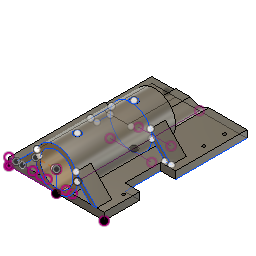
Pen Holder v2 (Autodesk Fusion 360 design; units mm, degrees)
Autodesk Fusion 360 part; units mm, degrees
sketch "Sketch1" plane through (0, 0, 0) normal (0, 1, 0) x (1, 0, 0)
  line L0 (0, 0) -> (32, 0)
  line L1 (32, 0) -> (32, 12)
  line L2 (32, 12) -> (27, 12)
  line L3 (27, 12) -> (27, 24)
  line L4 (27, 24) -> (32, 24)
  line L5 (32, 24) -> (32, 48)
  line L6 (32, 48) -> (0, 48)
  line L7 (0, 48) -> (0, 0)
  line L8 (0, 48) -> (16, 48)
  line L9 (16, 48) -> (16, 0)
  line L10 (0, 48) -> (5, 48)
  line L11 (8, 48) -> (8, 32)
  line L12 (8, 32) -> (0, 32)
  dimension "d1" = 32
  dimension "d2" = 12
  dimension "d3" = 12
  dimension "d4" = 24
  dimension "d5" = 16
  dimension "d6" = 5
  dimension "d7" = 16
  constraint coincident L0.start L7.end
  constraint horizontal L0
  constraint perpendicular L0 L1
  constraint horizontal L2
  constraint perpendicular L2 L3
  constraint perpendicular L3 L4
  constraint perpendicular L4 L5
  constraint perpendicular L5 L6
  constraint perpendicular L0 L7
  constraint coincident L6 L8.end
  constraint midpoint L0 L9.end
  constraint perpendicular L7 L10
  constraint midpoint L8 L11.start
  constraint perpendicular L8 L11
  constraint coincident L7 L12.end
  constraint perpendicular L7 L12
  measures "d1" distance of L0.start L0.end
  measures "d2" distance of L0.end L1.end
  measures "d3" distance of L2.end L3.end
  measures "d4" distance of L4.end L5.end
  measures "d5" distance of L6.end L8.end
  measures "d6" distance of L6.end L10.end
  measures "d7" distance of L11.start L11.end
extrude "Extrude1" add sketch "Sketch1" along normal blind 2.5 contours L0 L6 L7 L8 L9 L11 L12 | L0 L1 L2 L3 L4 L5 L6 L9 makes body 1
extrude "Extrude2" add sketch "Sketch1" along normal blind 2 contours L6 L7 L8 L10 L11 L12 bodies 1
sketch "Sketch2" plane through (0, 0, 0) normal (0, 0, 1) x (1, 0, 0)
  line L0 (32, 0) -> (0, 0)
  line L1 (32, 0) -> (16, 0)
  line L2 (0, 0) -> (32, 0)
  line L3 (0, 0) -> (32, 0)
  circle A0 centre (16, 7) radius 5.5
  circle A1 centre (16, 7) radius 7
  point P0 (32, 0)
  dimension "d12" = 16
  dimension "d14" = 11
  constraint coincident P0 L0.start
  constraint parallel L0 L1
  measures "d12" distance of P0 L1.end
  measures "d14" diameter of A0
extrude "Extrude3" cut sketch "Sketch2" against normal blind 53 contours A0 bodies 1
extrude "Extrude4" add sketch "Sketch2" against normal blind 33 bodies 1
sketch "Sketch3" plane through (0, 0, 0) normal (0, 0, 1) x (1, 0, 0)
  circle A0 centre (16, 7) radius 7
  line L0 (8, 2.5) -> (0, 2.5)
  line L1 (9.0003, 6.936) -> (4.5642, 2.5)
  line L2 (9.0003, 6.936) -> (15.2738, 6.936) construction
  line L3 (9.4734, 9.5304) -> (2.4429, 2.5)
  line L4 (7.9396, 7.9967) -> (10.1087, 7.9967) construction
  arc A1 (12.8377, 2.5) -> (19.1623, 2.5) centre (16, 7) ccw
  line L5 (16, 7) -> (16, 1.5)
  line L6 (22.5266, 9.5304) -> (29.5571, 2.5)
  line L7 (22.9997, 6.936) -> (27.4358, 2.5)
  line L8 (29.5571, 2.5) -> (27.4358, 2.5)
  line L9 (9.4734, 9.5304) -> (2.4429, 2.5)
  line L10 (9.0003, 6.936) -> (4.5642, 2.5)
  line L11 (9.4734, 9.5304) -> (2.4429, 2.5)
  line L12 (9.0003, 6.936) -> (4.5642, 2.5)
  line L13 (22.9997, 6.936, -25) -> (27.4358, 2.5, -25)
  line L14 (22.5266, 9.5304, -25) -> (29.5571, 2.5, -25)
  line L15 (9.4734, 9.5304, -25) -> (2.4429, 2.5, -25)
  line L16 (9.0003, 6.936, -25) -> (4.5642, 2.5, -25)
  line L17 (4.5642, 2.5, -25) -> (2.452, 2.5091, -25)
  line L18 (29.5571, 2.5, -25) -> (27.4358, 2.5, -25)
  circle A2 through (23, 7, -25) (12.5, 13.0622, -25) (12.5, 0.9378, -25)
  arc A3 (21.3619, 2.5) -> (10.6381, 2.5) centre (16, 7) ccw
  constraint coincident A0 L1.start
  constraint coincident L0 L1.end
  constraint coincident L4.start L3
  constraint coincident L0 L3.end
  constraint coincident A0.centre A1.centre
  constraint midpoint A1 L5.end
extrude "Extrude5" add sketch "Sketch3" against normal blind 5 contours A0 L0 L1 L3 L9 L10 L11 L12 A3 bodies 1
extrude "Extrude6" add sketch "Sketch3" against normal blind 5 contours A0 L6 L7 L8 A3 bodies 1
extrude "Extrude7" add sketch "Sketch3" against normal blind 5 separate body contours L13 L14 L18 A2 | L15 L16 L17 A2 in plane through (0, 0, -25) normal (0, 0, 1) makes body 2 at (7.1329, 7.19, -26.6667) makes body 3 at (24.8701, 7.187, -26.6667)
sketch "Sketch4" plane through (0, 0, 0) normal (0, 1, 0) x (1, 0, 0)
  line L0 (16, 48) -> (16, 0)
  line L1 (16, 0) -> (16, 7)
  circle A0 centre (16, 7) radius 1.25
  line L2 (10.5, 33) -> (21.5, 33)
  line L3 (9, 25) -> (23, 25)
  line L4 (16, 33) -> (16, 26)
  circle A1 centre (16, 26) radius 1.25
  circle A2 through (17.25, 26, 14) (15.375, 27.0825, 14) (15.375, 24.9175, 14)
  circle A3 through (17.25, 7, 14) (15.375, 8.0825, 14) (15.375, 5.9175, 14)
  point P0 (16, 0)
  dimension "d30" = 7
  dimension "d31" = 2.5
  dimension "d32" = 7
  dimension "d33" = 2.5
  constraint coincident P0 L0.end
  constraint coincident L0 L1.end
  constraint coincident L1.end A0.centre
  constraint midpoint L2 L4.start
  constraint perpendicular L3 L4
  constraint coincident L4.end A1.centre
  measures "d30" distance of P0 L1.end
  measures "d31" diameter of A0
  measures "d32" distance of L4.start L4.end
  measures "d33" diameter of A1
extrude "Extrude8" cut sketch "Sketch4" against normal blind 3 contours A2 | A3 in plane through (0, 14, 0) normal (0, 1, 0) bodies 1
sketch "Sketch7" plane through (0, 2.5, 0) normal (0, 1, 0) x (-1, 0, 0)
  line L0 (-27.4358, 0) -> (-27.4358, -5)
  line L1 (-27.4358, -5) -> (-29.5571, -5)
  line L2 (-29.5571, -5) -> (-29.5571, 0)
  line L3 (-29.5571, 0) -> (-32, 0)
  line L4 (-32, 0) -> (-32, -12)
  line L5 (-32, -12) -> (-27, -12)
  line L6 (-27, -12) -> (-27, -24)
  line L7 (-27, -24) -> (-32, -24)
  line L8 (-32, -24) -> (-32, -48)
  line L9 (-32, -48) -> (-19.1623, -48)
  line L10 (-19.1623, -48) -> (-19.1623, -33)
  line L11 (-19.1623, -33) -> (-21.3619, -33)
  line L12 (-21.3619, -33) -> (-21.3619, 0)
  line L13 (-21.3619, 0) -> (-27.4358, 0)
  line L14 (-32, -48) -> (-29.5, -48)
  line L15 (-29.5, -48) -> (-29.5, -43)
  circle A0 centre (-29.5, -43) radius 0.5
  line L16 (-32, -48) -> (0, -48)
  line L17 (-16, -48) -> (-16, -47)
  circle A1 centre (-2.5, -43) radius 0.5
  line L18 (-2.5, -43) -> (-2.5, -48)
  line L19 (-27, -18) -> (-2.5, -18)
  circle A2 centre (-2.5, -18) radius 0.5
  line L20 (-32, -12) -> (-29.5, -12)
  line L21 (-30.0678, -12) -> (-30.0678, -8.5)
  circle A3 centre (-30.0678, -8.5) radius 0.5
  line L22 (-30.0678, -8.5) -> (-2.5, -8.5)
  circle A4 centre (-2.5, -8.5) radius 0.5
  line L23 (-32, -48) -> (-32, -36)
  line L24 (-32, -36) -> (-29.5, -36)
  circle A5 centre (-29.5, -36) radius 0.5
  point P0 (-16, -48)
  dimension "d39" = 2.5
  dimension "d40" = 5
  dimension "d41" = 1
  dimension "d42" = 1
  dimension "d43" = 24.5
  dimension "d44" = 1
  dimension "d45" = 3.5
  dimension "d46" = 1
  dimension "d47" = 1
  dimension "d48" = 1
  constraint coincident L8.end L9.start
  constraint perpendicular L8 L14
  constraint perpendicular L14 L15
  constraint coincident L15.end A0.centre
  constraint coincident P0 L17.start
  constraint perpendicular L16 L17
  constraint symmetric A0 L17 A1
  constraint coincident A1.centre L18.start
  constraint coincident L16 L18.end
  constraint midpoint L6 L19.start
  constraint perpendicular L12 L19
  constraint coincident L19.end A2.centre
  constraint coincident L4.end L5.start
  constraint midpoint L5 L20.end
  constraint coincident L20 L21.start
  constraint perpendicular L20 L21
  constraint coincident L21.end A3.centre
  constraint parallel L19 L22
  constraint coincident L22.end A4.centre
  constraint midpoint L8 L23.end
  constraint perpendicular L23 L24
  constraint coincident L24.end A5.centre
  measures "d39" distance of L8.end L14.end
  measures "d40" distance of L14.end L15.end
  measures "d41" diameter of A0
  measures "d42" distance of P0 L17.end
  measures "d43" distance of L19.start L19.end
  measures "d44" diameter of A2
  measures "d45" distance of L21.start L21.end
  measures "d46" diameter of A3
  measures "d47" diameter of A4
  measures "d48" diameter of A5
extrude "Extrude9" cut sketch "Sketch7" against normal blind 5 contours L21 A3 L22 | L21 A3 L22 | A0 | A1 | A2 | A4 | A5 bodies 1
combine "Combine1" operation add target body 1 tool bodies 2 3
